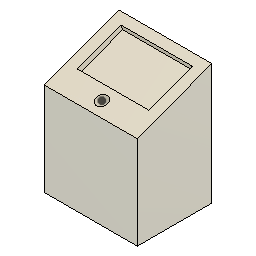
BOITIER INT v1 (Autodesk Fusion 360 design; units mm, degrees)
Autodesk Fusion 360 part; units mm, degrees
sketch "Sketch1" plane through (0, 0, 0) normal (0, 1, 0) x (1, 0, 0)
  line L0 (0, 0) -> (100, 0)
  line L1 (100, 0) -> (100, -80)
  line L2 (100, -80) -> (0, -80)
  line L3 (0, -80) -> (0, 0)
  dimension "d1" = 100
  dimension "d2" = 80
extrude "Extrude1" add sketch "Sketch1" along normal blind 130
sketch "Sketch2" plane through (100, 0, 0) normal (1, 0, 0) x (0, 0, -1)
  line L0 (-80, 0) -> (0, 0)
  line L1 (0, 0) -> (0, 130)
  line L2 (0, 130) -> (-80, 130)
  line L3 (-80, 130) -> (-80, 0)
  line L4 (-80, 130) -> (-80, 100)
  line L5 (-80, 100) -> (0, 130)
extrude "Extrude2" cut sketch "Sketch2" against normal blind 130 contours L2 L3 L4 L5
sketch "Sketch3" plane through (0, 113.9726, 42.7397) normal (0, 0.936329, 0.351123) x (1, 0, 0)
  line L0 (0, 45.646) -> (0, -39.794)
  line L1 (0, -39.794) -> (100, -39.794)
  line L2 (100, -39.794) -> (100, 45.646)
  line L3 (100, 45.646) -> (0, 45.646)
  line L4 (11.5, 35.646) -> (88.5, 35.646)
  line L5 (88.5, 35.646) -> (88.5, -14.354)
  line L6 (88.5, -14.354) -> (11.5, -14.354)
  line L7 (11.5, -14.354) -> (11.5, 35.646)
  circle A0 centre (50, -27.074) radius 6
  dimension "d7" = 50
  dimension "d8" = 77
  dimension "d9" = 11.5
  dimension "d10" = 19.8322
  dimension "d11" = 10
  dimension "d12" = 25.44
  dimension "d13" = 12.72
  dimension "d14" = 50
  dimension "d15" = 12
  measures "d8" distance of origin
  measures "d9" distance of L2 L5
  measures "d10" distance of L0 L7
  measures "d11" distance of L3 L4
  measures "d12" distance of L1 L6
  measures "d15" diameter of A0
extrude "Extrude4" cut sketch "Sketch3" against normal blind 40 contours A0
extrude "Extrude3" cut sketch "Sketch3" against normal blind 6 contours L4 L5 L6 L7
sketch "Sketch4" plane through (0, 0, 0) normal (0, 0, -1) x (-1, 0, 0)
  line L0 (-100, 0) -> (0, 0)
  line L1 (0, 0) -> (0, 130)
  line L2 (0, 130) -> (-100, 130)
  line L3 (-100, 130) -> (-100, 0)
  line L4 (-56.5, 11.5) -> (-53.5, 11.5)
  line L5 (-53.5, 11.5) -> (-53.5, 8.5)
  line L6 (-53.5, 8.5) -> (-56.5, 8.5)
  line L7 (-56.5, 8.5) -> (-56.5, 11.5)
  line L8 (-56.5, 11.5) -> (-53.5, 8.5) construction
  line L9 (-53.5, 11.5) -> (-56.5, 8.5) construction
  line L10 (-46.5, 11.5) -> (-43.5, 11.5)
  line L11 (-43.5, 11.5) -> (-43.5, 8.5)
  line L12 (-43.5, 8.5) -> (-46.5, 8.5)
  line L13 (-46.5, 8.5) -> (-46.5, 11.5)
  line L14 (-46.5, 11.5) -> (-43.5, 8.5) construction
  line L15 (-43.5, 11.5) -> (-46.5, 8.5) construction
  dimension "d20" = 10
  dimension "d21" = 10
  dimension "d22" = 3
  dimension "d23" = 3
  dimension "d24" = 3
  dimension "d25" = 3
  dimension "d30" = 45
extrude "Extrude7" cut sketch "Sketch4" against normal blind 20 contours L4 L5 L6 L7
extrude "Extrude5" cut sketch "Sketch4" against normal blind 14 contours L4 L5 L6 L7
extrude "Extrude6" cut sketch "Sketch4" against normal blind 18 contours L10 L11 L12 L13
equation "d13 = ( 25.44 / 2 ) * 1 mm"
